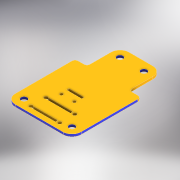
# Autodesk Inventor part: Base2
Saved by Autodesk Inventor 2021 (Build 250183000, 183)
## iProperties
Created: 2024-04-08
Part Number: Base2
Material: PLA
Document SubType Name: Modeling
Designer: Martin
Density: 1.27 g/cm^3
Appearance: PLA
Mass: 89.7051 g
Surface Area: 389.861 cm^2
Volume: 70.634 cm^3
Author: Martin
Autodesk Inventor part; units mm, degrees
ref_plane "YZ Plane" through (0, 0, 0) normal (1, 0, 0) x (0, 1, 0)
ref_plane "XZ Plane" through (0, 0, 0) normal (0, 1, 0) x (-1, 0, 0)
ref_plane "XY Plane" through (0, 0, 0) normal (0, 0, 1) x (1, 0, 0)
sketch "Sketch1" plane through (0, 0, 0) normal (0, 1, 0) x (-1, 0, 0)
  line L0 (-55, 85) -> (55, 85)
  line L1 (55, 85) -> (55, -85)
  line L2 (55, -85) -> (-55, -85)
  line L3 (-55, -85) -> (-55, 85)
  line L4 (-55, 85) -> (55, -85) construction
  line L5 (55, 85) -> (-55, -85) construction
  line L6 (77, 0) -> (-77, 0) projected
  line L7 (55, -85) -> (35, -85)
  line L8 (35, -85) -> (35, -30)
  line L9 (35, -30) -> (55, -30)
  line L10 (55, -30) -> (55, -85)
  line L11 (-55, -85) -> (-35, -85)
  line L12 (-35, -85) -> (-35, -30)
  line L13 (-35, -30) -> (-55, -30)
  line L14 (-55, -30) -> (-55, -85)
  point P0 (0, 0)
  dimension "d0" = 110
  dimension "d1" = 170
  dimension "d35" = 20
  dimension "d36" = 55
  dimension "d37" = 20
  dimension "d38" = 55
  constraints: 28 end point, 6 parallel, 3 horizontal, 3 perpendicular, 2 midpoint
  measures "d0" distance of L1.end L2.end
  measures "d1" distance of L0.end L1.end
  measures "d35" distance of L8.end L9.end
  measures "d36" distance of L7.end L8.end
  measures "d37" distance of L13.end L12.end
  measures "d38" distance of L12.end L11.end
extrude "Extrusion1" add sketch "Sketch1" along normal blind 4 contours L0 L1 L6 L3 | L6 L1 L9 L8 L2 L12 L13 L3
fillet "Fillet1" radius 15 2 edges at (-55, 2, 85) (55, 2, 85)
fillet "Fillet2" radius 15 2 edges at (-35, 2, -85) (35, 2, -85)
sketch "Sketch2" plane through (0, 4, 0) normal (0, 1, 0) x (1, 0, 0)
  line L0 (-55, 30) -> (-55, -70) projected
  arc A0 (-55, -70) -> (-40, -85) centre (-40, -70) ccw projected
  line L1 (-40, -85) -> (40, -85) projected
  arc A1 (40, -85) -> (55, -70) centre (40, -70) ccw projected
  line L2 (55, -70) -> (55, 30) projected
  line L3 (20, 85) -> (-20, 85) projected
  line L4 (55, 30) -> (35, 30) projected
  line L5 (35, 30) -> (35, 70) projected
  line L6 (-35, 70) -> (-35, 30) projected
  line L7 (-35, 30) -> (-55, 30) projected
  arc A2 (35, 70) -> (20, 85) centre (20, 70) ccw projected
  arc A3 (-20, 85) -> (-35, 70) centre (-20, 70) ccw projected
  point P0 (0, 0)
  point P1 (-4.3272, -2.2983)
  constraints: 4 coincident
hole "Hole1" at (40, 4, 70) at (-40, 4, 70) at (20, 4, -70) at (-20, 4, -70) direction (0, -1, 0) diameter 10 depth 4 tip angle 118
sketch "Sketch3" plane through (0, 4, 0) normal (0, 1, 0) x (1, 0, 0)
  line L0 (22.8472, -55) -> (-47.1528, -55)
  line L1 (-47.1528, -55) -> (-47.1528, 27)
  line L2 (-47.1528, 27) -> (22.8472, 27)
  line L3 (22.8472, 27) -> (22.8472, -55)
  line L4 (22.8472, -55) -> (-47.1528, 27) construction
  line L5 (-47.1528, -55) -> (22.8472, 27) construction
  line L6 (-40, -85) -> (40, -85) projected
  point P0 (0, 0)
  point P1 (-12.1528, -14)
  dimension "d12" = 70
  dimension "d13" = 82
  dimension "d34" = 30
  constraints: 12 end point, 2 midpoint, 2 parallel, 1 horizontal, 1 perpendicular
  measures "d12" distance of L1.end L2.end
  measures "d13" distance of L0.end L1.end
  measures "d34" distance between parallel lines of L6 L0
fillet "Fillet3" radius 5 4 edges at (-35, 2, -30) (-55, 2, -30) (55, 2, -30) (35, 2, -30)
sketch "Sketch5" plane through (0, 4, 0) normal (0, 1, 0) x (1, 0, 0)
  line L0 (-55, 12.5998) -> (-25, 12.5998)
  line L1 (-25, 12.5998) -> (-25, -27.4002)
  line L2 (-25, -27.4002) -> (-55, -27.4002)
  line L3 (-55, -27.4002) -> (-55, 12.5998)
  line L4 (0, -27.4002) -> (0, 4.9411)
  line L5 (-24, -76.5868) -> (24, -76.5868)
  line L6 (26, -74.5868) -> (26, -49.5868)
  line L7 (24, -47.5868) -> (-24, -47.5868)
  line L8 (-26, -49.5868) -> (-26, -74.5868)
  arc A0 (24, -76.5868) -> (26, -74.5868) centre (24, -74.5868) ccw
  arc A1 (-24, -47.5868) -> (-26, -49.5868) centre (-24, -49.5868) ccw
  arc A2 (26, -49.5868) -> (24, -47.5868) centre (24, -49.5868) ccw
  arc A3 (-26, -74.5868) -> (-24, -76.5868) centre (-24, -74.5868) ccw
  circle A4 centre (24, -74.5868) radius 3
  circle A5 centre (24, -49.5868) radius 3
  circle A6 centre (-24, -49.5868) radius 3
  circle A7 centre (-24, -74.5868) radius 3
  line L9 (-22, -76.5868) -> (19, -76.5868)
  line L10 (19, -76.5868) -> (19, -72.5868)
  line L11 (19, -72.5868) -> (-22, -72.5868)
  line L12 (-22, -72.5868) -> (-22, -76.5868)
  line L13 (26, -62.0868) -> (21, -62.0868)
  line L14 (19, -47.5868) -> (19, -51.5868)
  line L15 (19, -51.5868) -> (-22, -51.5868)
  line L16 (-22, -51.5868) -> (-22, -47.5868)
  line L17 (55, 12.5998) -> (25, 12.5998)
  line L18 (25, 12.5998) -> (25, -27.4002)
  line L19 (25, -27.4002) -> (55, -27.4002)
  line L20 (5.6733, -33.7631) -> (-15.8267, -33.7631)
  line L21 (-17.8267, -31.7631) -> (-17.8267, -18.2631)
  line L22 (-17.8267, -18.2631) -> (7.6733, -18.2631)
  line L23 (7.6733, -18.2631) -> (7.6733, -31.7631)
  arc A8 (-17.8267, -31.7631) -> (-15.8267, -33.7631) centre (-15.8267, -31.7631) ccw
  arc A9 (-17.8267, -31.7631) -> (-15.8267, -33.7631) centre (-15.8267, -31.7631) ccw
  arc A10 (5.6733, -33.7631) -> (7.6733, -31.7631) centre (5.6733, -31.7631) ccw
  circle A11 centre (-15.8267, -31.7631) radius 2.5
  circle A12 centre (5.6733, -31.7631) radius 2.5
  line L24 (-17.8267, -18.2631) -> (7.6733, -18.2631)
  line L25 (7.6733, -18.2631) -> (7.6733, -21.2631)
  line L26 (7.6733, -21.2631) -> (-17.8267, -21.2631)
  line L27 (-17.8267, -21.2631) -> (-17.8267, -18.2631)
  line L28 (-17.8267, -18.2631) -> (7.6733, -18.2631)
  line L29 (7.6733, -18.2631) -> (7.6733, -17.2631)
  line L30 (7.6733, -17.2631) -> (-17.8267, -17.2631)
  line L31 (-17.8267, -17.2631) -> (-17.8267, -18.2631)
  point P0 (0, 0)
  point P1 (26, -47.5868)
  point P2 (26, -76.5868)
  point P3 (-26, -47.5868)
  point P4 (-17.8267, -33.7631)
  point P5 (-21.7639, -47.5868)
  point P6 (-21.7639, -51.5868)
  point P7 (-21.7639, -72.5868)
  point P8 (-21.7639, -76.5868)
  point P9 (19, -76.5868)
  dimension "d41" = 30
  dimension "d42" = 40
  dimension "d43" = 52
  dimension "d44" = 29
  dimension "d45" = 2
  dimension "d46" = 6
  dimension "d47" = 6
  dimension "d48" = 6
  dimension "d49" = 6
  dimension "d50" = 4
  dimension "d51" = 41
  dimension "d52" = 7
  dimension "d53" = 25.5
  dimension "d54" = 15.5
  dimension "d55" = 2
  dimension "d56" = 5
  dimension "d57" = 5
  dimension "d62" = 3
  dimension "d63" = 1
  constraints: 64 end point, 14 point on circle, 14 tangent, 13 centre point, 12 parallel, 12 point on line, 8 symmetric about line, 7 horizontal, 6 coincident, 6 perpendicular, 5 equal radius, 1 midpoint, 1 vertical, 1 other
  measures "d41" distance of L1.end L2.end
  measures "d42" distance of L0.end L1.end
  measures "d43" distance of point (-26, -47.587) point (26, -47.587)
  measures "d44" distance of point (26, -47.587) point (26, -76.587)
  measures "d45" radius of A0
  measures "d46" diameter of A4
  measures "d47" diameter of A5
  measures "d48" diameter of A6
  measures "d49" diameter of A7
  measures "d50" distance of L10.end L9.end
  measures "d51" distance of L10.end L11.end
  measures "d52" distance between parallel lines of L10 L6
  measures "d53" distance of L21.end L22.end
  measures "d54" distance of point (-17.827, -33.763) L21.end
  measures "d55" radius of A8
  measures "d56" diameter of A11
  measures "d57" diameter of A12
  measures "d62" distance of L24.end L25.end
  measures "d63" distance of L29.end L28.end
extrude "Extrusion3" cut sketch "Sketch5" against normal up to next contours L26 L21 L22 L4 | L4 L22 L23 L26 | L22 L31 L30 L4 | L4 L30 L29 L22 | A12 L20 A10 L23 | L23 A10 L20 A12 | A11 L20 A8 L21 | L21 A8 L20 A11 | A3 L8 A7 L11 L12 L5 | L5 A7 L8 A3 | L12 L11 A7 L5 | A7 L11 L10 L5 | A6 L7 A1 L8 | L8 A1 L7 L16 L15 A6 | A4 L6 A0 L5 | L5 A0 L6 A4 | A6 L15 L16 L7 | L7 L14 L15 A6 | A5 L6 A2 L7 | L7 A2 L6 A5
body "Solid1"
